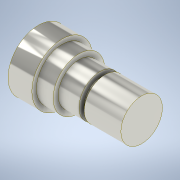
# Autodesk Inventor part: lab_4_1
Saved by Autodesk Inventor 2020 (Build 240168000, 168)
## iProperties
Created: 2020-03-17
Part Number: lab_4_1
Material: Серебро
Document SubType Name: Modeling
Designer: User
Density: 10.49 g/cm^3
Appearance: Серебро
Author: User
Autodesk Inventor part; units mm, degrees
ref_plane "YZ Plane" through (0, 0, 0) normal (1, 0, 0) x (0, 1, 0)
ref_plane "XZ Plane" through (0, 0, 0) normal (0, 1, 0) x (-1, 0, 0)
ref_plane "XY Plane" through (0, 0, 0) normal (0, 0, 1) x (1, 0, 0)
sketch "Эскиз1" plane through (0, 0, 0) normal (0, 0, 1) x (1, 0, 0)
  line L0 (0, 0) -> (100, 0)
  line L1 (100, 0) -> (100, 20.0896)
  line L2 (100, 20.0896) -> (39.2522, 20.0896)
  line L3 (39.2522, 20.0896) -> (39.2522, 24.9514)
  line L4 (39.2522, 24.9514) -> (23.0464, 24.9514)
  line L5 (23.0464, 24.9514) -> (23.0464, 29.3145)
  line L6 (23.0464, 29.3145) -> (0, 29.3145)
  line L7 (0, 29.3145) -> (0, 0)
  line L8 (59.4742, 20.0896) -> (59.4742, 15.0896)
  line L9 (59.4742, 15.0896) -> (64.4742, 15.0896)
  line L10 (64.4742, 15.0896) -> (64.4742, 20.0896)
  dimension "d0" = 100
  dimension "d2" = 5
  dimension "d3" = 5
  constraints: 22 end point, 9 perpendicular, 2 point on line, 1 horizontal, 1 vertical
  measures "d0" distance of L0.start L0.end
  measures "d2" distance of L8.start L8.end
  measures "d3" distance of L8.end L9.end
revolve "Вращение1" add sketch "Эскиз1" angle 360 about axis through (0, 0, 0) along (1, 0, 0)
revolve "Вращение2" add sketch "Эскиз1" angle 360 about axis through (0, 0, 0) along (1, 0, 0) contours L10 L9 L8 L2
revolve "Вращение3" cut sketch "Эскиз1" angle 360 mid plane about axis through (0, 0, 0) along (1, 0, 0) contours L10 L9 L8 L2
